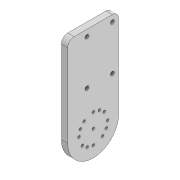
# Autodesk Inventor part: StereoVisionHolder_2
Saved by Autodesk Inventor 2022 (Build 260153000, 153)
## iProperties
Created: 2022-11-13
Part Number: StereoVisionHolder_2
Material: Generic
Document SubType Name: Modeling
Designer: MVeszpremi
Density: 1 g/cm^3
Appearance: Default
Author: MVeszpremi
Autodesk Inventor part; units mm, degrees
ref_plane "YZ Plane" through (0, 0, 0) normal (1, 0, 0) x (0, 1, 0)
ref_plane "XZ Plane" through (0, 0, 0) normal (0, 1, 0) x (-1, 0, 0)
ref_plane "XY Plane" through (0, 0, 0) normal (0, 0, 1) x (1, 0, 0)
sketch "Sketch2" plane through (0, 0, 0) normal (1, 0, 0) x (0, 1, 0)
  circle A0 centre (0, 0) radius 11.25
  circle A1 centre (11.25, 0) radius 1
  circle A2 centre (0, 11.25) radius 1
  circle A3 centre (-11.25, 0) radius 1
  circle A4 centre (0, -11.25) radius 1
  circle A5 centre (7.2314, -8.618) radius 1
  line L0 (0, 0) -> (7.2314, -8.618)
  line L1 (0, 0) -> (11.25, 0)
  circle A6 centre (8.618, 7.2314) radius 1
  circle A7 centre (-7.2314, 8.618) radius 1
  circle A8 centre (-8.618, -7.2314) radius 1
  circle A9 centre (10.196, -4.7545) radius 1
  line L2 (0, 0) -> (10.196, -4.7545)
  circle A10 centre (4.7545, 10.196) radius 1
  circle A11 centre (-10.196, 4.7545) radius 1
  circle A12 centre (-4.7545, -10.196) radius 1
  circle A13 centre (0, 0) radius 20
  line L3 (0, 20) -> (70, 20)
  line L4 (70, 20) -> (70, -20)
  line L5 (70, -20) -> (0, -20)
  line L6 (0, -20) -> (0, 20)
  line L7 (70, 20) -> (0, 20)
  line L8 (0, 20) -> (0, 15)
  line L9 (0, 15) -> (70, 15)
  line L10 (70, 15) -> (70, 20)
  circle A14 centre (0, 0) radius 1
  point P0 (13.2288, 15)
  dimension "d0" = 22.5
  dimension "d1" = 2
  dimension "d4" = 360
  dimension "d6" = 2
  dimension "d7" = 50
  dimension "d10" = 360
  dimension "d12" = 2
  dimension "d13" = 25
  dimension "d16" = 360
  dimension "d18" = 40
  dimension "d19" = 70
  dimension "d20" = 5
  dimension "d21" = 2
  constraints: 22 end point, 15 centre point, 5 point on circle, 4 parallel, 3 coincident, 3 horizontal, 2 perpendicular, 1 point on line, 27 other
  measures "d0" diameter of A0
  measures "d1" diameter of A1
  measures "d6" diameter of A5
  measures "d7" angle of L0 L1
  measures "d12" diameter of A9
  measures "d13" angle of L1 L2
  measures "d18" diameter of A13
  measures "d19" distance of L4.end L5.end
  measures "d20" distance between parallel lines of L7 L9
  measures "d21" diameter of A14
extrude "Extrusion1" add sketch "Sketch2" along normal blind 5 contours A1 L1 A14 L6 A2 A0 A10 A6 | A0 A6 A10 A2 L6 L9 A13 A4 A5 A9 A1 | A0 A9 L2 A14 L1 A1 | A9 A0 A5 L0 A14 L2 | A14 L6 A4 A0 A12 A8 A3 A11 A7 A2 | L0 A5 A0 A4 L6 A14 | A0 A7 A11 A3 A8 A12 A4 L6 A13 A2 | L6 A13 L9 | A13 L9 L4 L5 | L3 L4 L9 A13
sketch "Sketch3" plane through (5, 0, 0) normal (1, 0, 0) x (0, 0, -1)
  circle A0 centre (-5, 65) radius 1.5
  line L0 (20, 70) -> (-20, 70) projected
  line L1 (-20, 70) -> (-20, 0) projected
  circle A1 centre (15, 65) radius 1.5
  circle A2 centre (-5, 30) radius 1.5
  circle A3 centre (15, 30) radius 1.5
  point P0 (0, 0)
  dimension "d24" = 5
  dimension "d25" = 15
  dimension "d26" = 3
  dimension "d29" = 20
  dimension "d32" = 35
  constraints: 4 centre point, 1 horizontal, 1 vertical, 6 other
  measures "d24" distance from line of L0 A0.centre
  measures "d25" distance from line of L1 A0.centre
  measures "d26" diameter of A0
  measures "d29" distance of A0.centre A1.centre
  measures "d32" distance of A0.centre A2.centre
extrude "Extrusion2" cut sketch "Sketch3" against normal blind 5
fillet "Fillet1" radius 5 2 edges at (2.5, 70, 20) (2.5, 70, -20)
body "Solid1"
